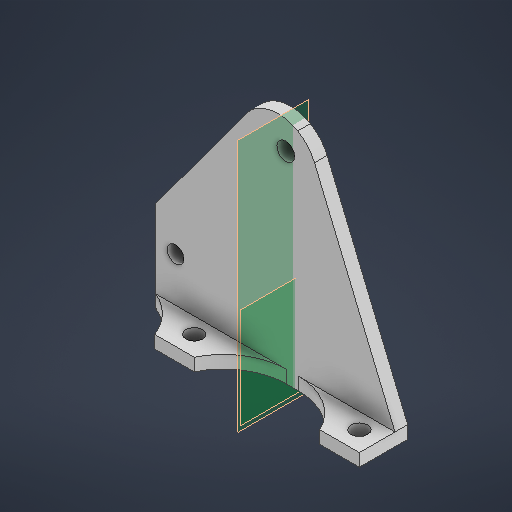
# Autodesk Inventor part: мертвое колесо 3
Saved by Autodesk Inventor 2026.2 (Build 302298000, 298)
## iProperties
Created: 2025-09-25
Part Number: мертвое колесо 3
Material: Типовые
Document SubType Name: Modeling
Designer: GameHD
Density: 1 g/cm^3
Appearance: По умолчанию
Author: GameHD
Autodesk Inventor part; units mm, degrees
ref_plane "YZ Plane" through (0, 0, 0) normal (1, 0, 0) x (0, 1, 0)
ref_plane "XZ Plane" through (0, 0, 0) normal (0, 1, 0) x (-1, 0, 0)
ref_plane "XY Plane" through (0, 0, 0) normal (0, 0, 1) x (1, 0, 0)
sketch "Эскиз1" plane through (0, 0, 0) normal (0, 0, 1) x (1, 0, 0)
  circle A0 centre (0, 0) radius 2.1
  line L0 (-5, 14.35) -> (5, 14.35)
  line L1 (5, 14.35) -> (5, -14.35)
  line L2 (5, -14.35) -> (-5, -14.35)
  line L3 (-5, -14.35) -> (-5, 14.35)
  line L4 (-5, 14.35) -> (5, -14.35) construction
  line L5 (5, 14.35) -> (-5, -14.35) construction
  line L6 (-5, 7) -> (5, 7)
  dimension "d0" = 4.2
  dimension "d2" = 10
  dimension "d3" = 28.7
  dimension "d4" = 7
  constraints: 14 end point, 2 midpoint, 2 parallel, 2 perpendicular, 2 point on line, 1 centre point, 1 coincident, 1 horizontal
  measures "d0" diameter of A0
  measures "d2" distance of L1.end L2.end
  measures "d3" distance of L2.end L0.start
  measures "d4" distance from line of A0.centre L6
extrude "Выдавливание1" add sketch "Эскиз1" along normal blind 3.2 contours L6 L1 L2 L3
sketch "Эскиз2" plane through (0, 0, 3.2) normal (0, 0, 1) x (1, 0, 0)
  line L0 (5, -14.35) -> (5, 7) projected
  line L1 (5, -14.35) -> (-5, -14.35)
  line L2 (-5, -14.35) -> (-5, -11.15)
  line L3 (-5, -11.15) -> (5, -11.15)
  line L4 (5, -11.15) -> (5, -14.35)
  point P0 (0, 0)
  point P1 (5, -11.15)
  dimension "d7" = 10
  dimension "d8" = 3.2
  constraints: 8 end point, 2 parallel, 1 horizontal, 1 perpendicular
  measures "d7" distance of L2.end L3.end
  measures "d8" distance of L1.end L2.end
extrude "Выдавливание2" add sketch "Эскиз2" along normal blind 13
sketch "Эскиз3" plane through (-5, -11.15, 16.2) normal (0, 1, 0) x (1, 0, 0)
  line L0 (0, 10) -> (10, 10) projected
  line L1 (5, 10) -> (5, 0)
  line L2 (0, 0) -> (10, 0) projected
  circle A0 centre (5, 5) radius 2.1
  point P0 (5, 16.2)
  dimension "d12" = 4.2
  constraints: 3 midpoint, 2 end point, 1 centre point
  measures "d12" diameter of A0
extrude "Выдавливание3" cut sketch "Эскиз3" against normal blind 13
sketch "Эскиз4" plane through (0, 0, 3.2) normal (0, 0, 1) x (1, 0, 0)
  circle A0 centre (27.823512, 36.442015) radius 2.691667
  line L0 (25.598764, 34.926903) -> (0, 0)
  line L1 (17.757888, 39.624709) -> (-5, 8.573892)
  line L2 (-5, 7) -> (-5, -11.15)
  line L3 (-5, 7) -> (-5, 8.573892)
  line L4 (-5, -14.35) -> (5, -14.35)
  line L5 (5, -14.35) -> (5, -11.15)
  line L6 (5, -11.15) -> (-5, -11.15)
  line L7 (-5, -11.15) -> (-5, -14.35)
  line L8 (27.823512, 36.442015) -> (27.823512, -3.381482)
  line L9 (35.823512, 33.713219) -> (35.823512, -14.35)
  arc A1 (35.823512, 33.713219) -> (17.757888, 39.624709) centre (25.823512, 33.713219) ccw
  line L10 (-5, -14.35) -> (35.823512, -14.35)
  circle A2 centre (27.823512, 36.442015) radius 2.25
  line L11 (-5, 8.573892) -> (-5, -14.35)
  circle A3 centre (0, 0) radius 2.1
  point P0 (-5, -8.15)
  point P1 (-5, -11.15)
  dimension "d15" = 10
  dimension "d16" = 8
  dimension "d17" = 10
  dimension "d18" = 4.5
  constraints: 14 end point, 2 centre point, 2 parallel, 2 point on circle, 2 tangent, 2 vertical, 1 coincident, 1 horizontal, 1 perpendicular, 2 other
  measures "d15" distance from line of L8.start L1
  measures "d16" distance between parallel lines of L8 L9
  measures "d17" radius of A1
  measures "d18" diameter of A2
extrude "Выдавливание4" add sketch "Эскиз4" against normal up to surface (3.2 mm away) contours A0 | A1 L9 L10 L5 L6 L2 L3 L1
ref_plane "РабПлоскость1" through (20.202, -14.35, 16.2) normal (-1, 0, 0) x (0, 0, 1)
mirror "Зеркальное отражение1" about plane through (20.202, -14.35, 16.2) normal (-1, 0, 0) of "Выдавливание2", "Выдавливание3"
sketch "Эскиз6" plane through (0, 0, 0) normal (0, 0, -1) x (-1, 0, 0)
  circle A0 centre (-17.823512, 36.442015) radius 2.25
  circle A1 centre (10, 0) radius 2.1
  line L0 (5, -14.35) -> (-35.823512, -14.35)
  line L1 (5, -14.35) -> (5, 8.573892)
  line L2 (15, 8.573892) -> (-7.757888, 39.624709)
  arc A2 (-7.757888, 39.624709) -> (-25.823512, 33.713219) centre (-15.823512, 33.713219) ccw
  line L3 (-25.823512, 33.713219) -> (-25.823512, -14.35)
  circle A3 centre (-27.823512, 36.442015) radius 2.25
  circle A4 centre (0, 0) radius 2.1
  line L4 (5, -14.35) -> (-35.823512, -14.35)
  line L5 (5, -14.35) -> (5, 8.573892)
  line L6 (5, 8.573892) -> (-17.757888, 39.624709)
  arc A5 (-17.757888, 39.624709) -> (-35.823512, 33.713219) centre (-25.823512, 33.713219) ccw
  line L7 (-35.823512, 33.713219) -> (-35.823512, -14.35)
  line L8 (-35.823512, -14.35) -> (-35.823512, -11.15)
  line L9 (-35.823512, -11.15) -> (-45.404, -11.15)
  line L10 (-45.404, -11.15) -> (-45.404, -14.35)
  line L11 (-45.404, -14.35) -> (-35.823512, -14.35)
  line L12 (-25.823512, -14.35) -> (-45.404, -14.35)
  line L13 (0, 0) -> (10, 0)
  line L14 (15, 8.573892) -> (15, -18.0489)
  line L15 (-5, -14.35) -> (-35.404, -14.35)
  line L16 (-8, -14.35) -> (16.577235, -14.35)
  line L17 (-45.404, -11.15) -> (-35.708646, 35.224555)
  point P0 (-10, 0)
  point P1 (-20.823512, 42.373473)
  point P2 (15, -14.35)
  point P3 (-16.942673, 38.512431)
  point P4 (-15.583961, 36.658607)
  point P5 (5, 8.573892)
  dimension "d35" = 10
  constraints: 14 end point, 5 centre point, 3 point on circle, 2 horizontal, 1 perpendicular, 1 vertical
  measures "d35" distance of L13.start L13.end
extrude "Выдавливание5" add sketch "Эскиз6" against normal up to surface (3.2 mm away) contours A0 L6 A5 A2 L2 L14 L16 L1 | A5 L7 L9 L17 | L9 L7 L11 L10
extrude "Выдавливание6" cut sketch "Эскиз6" against normal blind 10 contours A0 L6 | L6 A0 | A1
sketch "Эскиз7" plane through (0, 0, 3.2) normal (0, 0, 1) x (1, 0, 0)
  circle A0 centre (0, 0) radius 2.1
  line L0 (35.404, -14.35) -> (35.404, -11.15)
  line L1 (5, -14.35) -> (35.404, -14.35)
  arc A1 (35.708646, 35.224555) -> (20.823512, 42.373473) centre (25.823512, 33.713219) ccw
  line L2 (30.823512, 42.373473) -> (-5, -8.15)
  line L3 (35.404, -11.15) -> (45.404, -11.15)
  arc A2 (20.823512, 42.373473) -> (7.757888, 39.624709) centre (15.823512, 33.713219) ccw
  line L4 (-15, 8.573892) -> (7.757888, 39.624709)
  line L5 (-15, -14.35) -> (-15, 8.573892)
  line L6 (-5, -14.35) -> (-15, -14.35)
  line L7 (-5, -11.15) -> (-5, -14.35)
  circle A3 centre (17.823512, 36.442015) radius 2.25
  circle A4 centre (17.823512, 36.442015) radius 2.25
  circle A5 centre (27.823512, 36.442015) radius 2.25
  circle A6 centre (0, 0) radius 2.1
  circle A7 centre (-10, 0) radius 2.1
  line L8 (5, -14.35) -> (35.404, -14.35)
  line L9 (35.404, -14.35) -> (35.404, -11.15)
  line L10 (35.404, -11.15) -> (45.404, -11.15)
  arc A8 (35.708646, 35.224555) -> (20.823512, 42.373473) centre (25.823512, 33.713219) ccw
  arc A9 (20.823512, 42.373473) -> (7.757888, 39.624709) centre (15.823512, 33.713219) ccw
  line L11 (-15, 8.573892) -> (7.757888, 39.624709)
  line L12 (-15, -14.35) -> (-15, 8.573892)
  line L13 (-5, -14.35) -> (-15, -14.35)
  line L14 (-5, -11.15) -> (-5, -14.35)
  line L15 (35.708646, 35.224555) -> (45.404, -11.15)
  line L16 (35.708646, 35.224555) -> (45.404, -11.15)
  circle A10 centre (15.823537, 33.690994) radius 10.021745
  circle A11 centre (25.823512, 33.713219) radius 10
  line L17 (35.708646, 35.224555) -> (-5, 35.224555)
  line L18 (45.404, -11.15) -> (25.071691, 37.551955)
  line L19 (5, -14.35) -> (5, -11.15)
  line L20 (5, -14.35) -> (5, -11.15)
  line L21 (-5, -11.15) -> (5, -11.15)
  line L22 (-5, -11.15) -> (5, -11.15)
  point P0 (-0.639537, -2.000248)
  point P1 (1.675949, 1.265384)
  point P2 (20.826018, 42.374919)
  constraints: 6 end point, 1 centre point, 1 coincident, 1 concentric, 1 horizontal, 4 other
extrude "Выдавливание7" add sketch "Эскиз7" against normal up to surface (3.2 mm away) contours A0 L2 | L2 A0 | L17 L18 L2 A5 | A5 L18 L17 | A5 L17 L18 | L2 L18 A5 | L17 A5 L2 L18 | L2 A5 L18
sketch "Эскиз7 outline for Выдавливание8" plane through (0, 0, 3.2) normal (0, 0, 1) x (1, 0, 0)
  arc A0 (35.708646, 35.224555) -> (20.826018, 42.374919) centre (25.823512, 33.713219) ccw
  line L0 (45.404, -11.15) -> (35.708646, 35.224555)
  line L1 (25.071691, 37.551955) -> (45.404, -11.15)
  arc A1 (20.826018, 42.374919) -> (25.071691, 37.551955) centre (15.823537, 33.690994) cw
extrude "Выдавливание8" cut sketch "Эскиз7 outline for Выдавливание8" against normal blind 10
sketch "Эскиз9" plane through (-5, -11.15, 16.2) normal (0, 1, 0) x (1, 0, 0)
  circle A0 centre (3.712, 5) radius 2.1
  line L0 (-1.288, 10) -> (8.712, 10)
  line L1 (-1.288, 10) -> (-1.288, 0)
  line L2 (8.712, 0) -> (-1.288, 0)
  line L3 (8.712, 13) -> (8.712, 0)
  line L4 (50.404, 13) -> (30.071691, 13)
  line L5 (30.071691, 13) -> (25.826018, 13)
  line L6 (25.826018, 13) -> (25.823512, 13)
  line L7 (12.757888, 13) -> (25.823512, 13)
  line L8 (-10, 13) -> (12.757888, 13)
  line L9 (0, 13) -> (-10, 13)
  line L10 (10, 13) -> (40.404, 13)
  line L11 (25.073512, 13) -> (20.573512, 13)
  line L12 (-7.1, 13) -> (-2.9, 13)
  line L13 (-1.288, 10) -> (-1.288, 15.274869)
  line L14 (0, 13) -> (0, 0)
  line L15 (0, 13) -> (0, 0)
  circle A1 centre (5, 5) radius 2.1
  line L16 (0, 13) -> (0, 0)
  line L17 (10, 0) -> (0, 0)
  line L18 (10, 13) -> (10, 0)
  line L19 (0, 13) -> (10, 13)
  line L20 (0, 13) -> (10, 13)
  line L21 (8.712, 10) -> (12.757888, 10)
  line L22 (3.712, 5) -> (3.712, 9)
  circle A2 centre (3.712, 9) radius 2.1
  line L23 (11.441296, 4) -> (-2.9, 4)
  line L24 (40.404, 13) -> (50.404, 13)
  point P0 (5, 16.2)
  point P1 (0, 10)
  point P2 (-1.288, 13)
  point P3 (0, 10)
  point P4 (-1.288, 4)
  point P5 (8.712, 4)
  dimension "d42" = 4
  dimension "d43" = 4.2
  dimension "d44" = 4
  constraints: 16 end point, 3 centre point, 2 horizontal, 2 point on line, 2 vertical, 1 coincident
  measures "d42" distance of L22.start L22.end
  measures "d43" diameter of A2
  measures "d44" distance between parallel lines of L23 L17
extrude "Выдавливание10" add sketch "Эскиз9" against normal up to surface (3.2 mm away) contours A0 L23 A1 | A0 A1 L23 | A1 L22 A2 A0 | A0 A2 L0 L3 L23 A1 | L23 A1 A0 | A0 A1 L23 | A2 L22 A0 | A0 A2 L0 | A1 L23 A0 A2 L22 | A1 L23 L3 L2 L14 A0 | A0 L23 A1 | L22 A2 A0 | L23 L14 L0 A2 A0 | L23 L1 L0 L14 | L14 L2 L1 L23 | L0 L13 L8 L14
extrude "Выдавливание11" cut sketch "Эскиз9" against normal blind 10 contours L23 A1 A0 | A0 A1 L23 | A2 L22 A0 | A0 A2 L0 | A1 L23 L3 L2 L14 A0 | A0 L23 A1 | L22 A2 A0 | L23 L18 L17 L3 | L3 L21 L18 L23 | L0 A2 | L14 L2 L1 L23 | L3 L8 L18 L21 picked at (6.324605, 3.867911) picked at (4.682533, 3.889371) picked at (2.387395, 3.867911)
ref_plane "РабПлоскость2" through (19.558, -14.35, 16.2) normal (-1, 0, 0) x (0, 0, 1)
mirror "Зеркальное отражение2" about plane through (19.558, -14.35, 16.2) normal (-1, 0, 0) of "Выдавливание11", "Выдавливание10"
fillet "Сопряжение5" radius 16 3 edges at (35.404, -12.75, 3.2) (3.712, -12.75, 3.2) (-6.288, -12.75, 3.2)
